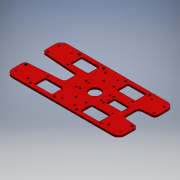
# Autodesk Inventor part: top_plate
Saved by Autodesk Inventor 2016 (Build 200138000, 138)
## iProperties
Created: 2015-12-08
Part Number: top_plate
Material: Generic
Document SubType Name: Modeling
Designer: lk8187
Density: 1 g/cm^3
Appearance: Smooth - Burnt Red
Author: lk8187
Autodesk Inventor part; units mm, degrees
ref_plane "YZ Plane" through (0, 0, 0) normal (1, 0, 0) x (0, 1, 0)
ref_plane "XZ Plane" through (0, 0, 0) normal (0, 1, 0) x (-1, 0, 0)
ref_plane "XY Plane" through (0, 0, 0) normal (0, 0, 1) x (1, 0, 0)
sketch "Sketch1" plane through (0, 0, 0) normal (0, 0, 1) x (1, 0, 0)
  line L0 (138.5, 75.5) -> (138.5, 61)
  arc A0 (136.5, 59) -> (138.5, 61) centre (136.5, 61) ccw
  line L1 (136.5, 59) -> (110, 59)
  arc A1 (108, 61) -> (110, 59) centre (110, 61) ccw
  line L2 (108, 61) -> (108, 75.5)
  arc A2 (110, 77.5) -> (108, 75.5) centre (110, 75.5) ccw
  line L3 (110, 77.5) -> (136.5, 77.5)
  arc A3 (138.5, 75.5) -> (136.5, 77.5) centre (136.5, 75.5) ccw
  line L4 (62, 75.5) -> (62, 61)
  arc A4 (60, 59) -> (62, 61) centre (60, 61) ccw
  line L5 (60, 59) -> (35, 59)
  arc A5 (33, 61) -> (35, 59) centre (35, 61) ccw
  line L6 (33, 61) -> (33, 75.5)
  arc A6 (35, 77.5) -> (33, 75.5) centre (35, 75.5) ccw
  line L7 (35, 77.5) -> (60, 77.5)
  arc A7 (62, 75.5) -> (60, 77.5) centre (60, 75.5) ccw
  line L8 (62, 17) -> (62, 2.5)
  arc A8 (60, 0.5) -> (62, 2.5) centre (60, 2.5) ccw
  line L9 (60, 0.5) -> (35, 0.5)
  arc A9 (33, 2.5) -> (35, 0.5) centre (35, 2.5) ccw
  line L10 (33, 2.5) -> (33, 17)
  arc A10 (35, 19) -> (33, 17) centre (35, 17) ccw
  line L11 (35, 19) -> (60, 19)
  arc A11 (62, 17) -> (60, 19) centre (60, 17) ccw
  line L12 (138.5, 17) -> (138.5, 2.5)
  arc A12 (136.5, 0.5) -> (138.5, 2.5) centre (136.5, 2.5) ccw
  line L13 (136.5, 0.5) -> (110, 0.5)
  arc A13 (108, 2.5) -> (110, 0.5) centre (110, 2.5) ccw
  line L14 (108, 2.5) -> (108, 17)
  arc A14 (110, 19) -> (108, 17) centre (110, 17) ccw
  line L15 (110, 19) -> (136.5, 19)
  arc A15 (138.5, 17) -> (136.5, 19) centre (136.5, 17) ccw
  arc A16 (176, 19.861) -> (171.3739, 24.847) centre (171, 19.861) ccw
  line L16 (171.3739, 24.847) -> (155.6261, 26.028)
  arc A17 (151, 31.014) -> (155.6261, 26.028) centre (156, 31.014) ccw
  line L17 (151, 31.014) -> (151, 46.986)
  arc A18 (155.6261, 51.972) -> (151, 46.986) centre (156, 46.986) ccw
  line L18 (155.6261, 51.972) -> (171.3739, 53.153)
  arc A19 (171.3739, 53.153) -> (176, 58.139) centre (171, 58.139) ccw
  line L19 (176, 58.139) -> (176, 73.5)
  arc A20 (176, 73.5) -> (166, 83.5) centre (166, 73.5) ccw
  line L20 (166, 83.5) -> (4, 83.5)
  arc A21 (4, 83.5) -> (-6, 73.5) centre (4, 73.5) ccw
  line L21 (-6, 73.5) -> (-6, 58.139)
  arc A22 (-6, 58.139) -> (-1.3739, 53.153) centre (-1, 58.139) ccw
  line L22 (-1.3739, 53.153) -> (49.3739, 49.347)
  arc A23 (54, 44.361) -> (49.3739, 49.347) centre (49, 44.361) ccw
  line L23 (54, 44.361) -> (54, 33.639)
  arc A24 (49.3739, 28.653) -> (54, 33.639) centre (49, 33.639) ccw
  line L24 (49.3739, 28.653) -> (-1.3739, 24.847)
  arc A25 (-1.3739, 24.847) -> (-6, 19.861) centre (-1, 19.861) ccw
  line L25 (-6, 19.861) -> (-6, 4.5)
  arc A26 (-6, 4.5) -> (4, -5.5) centre (4, 4.5) ccw
  line L26 (4, -5.5) -> (166, -5.5)
  arc A27 (166, -5.5) -> (176, 4.5) centre (166, 4.5) ccw
  line L27 (176, 4.5) -> (176, 19.861)
  line L28 (118.205, 45.5) -> (142.275, 45.5)
  line L29 (142.275, 45.5) -> (142.275, 32.5)
  line L30 (142.275, 32.5) -> (118.205, 32.5)
  line L31 (118.205, 32.5) -> (118.205, 45.5)
  circle A28 centre (150, 4) radius 1.5
  circle A29 centre (170, 74) radius 1.5
  circle A30 centre (75, 74) radius 1.5
  circle A31 centre (20, 74) radius 1.5
  circle A32 centre (0, 4) radius 1.5
  circle A33 centre (95, 4) radius 1.5
  circle A34 centre (0, 74) radius 1.5
  circle A35 centre (20, 4) radius 1.5
  circle A36 centre (75, 4) radius 1.5
  circle A37 centre (95, 74) radius 1.5
  circle A38 centre (150, 74) radius 1.5
  circle A39 centre (170, 4) radius 1.5
  circle A40 centre (93, 39) radius 9
  circle A41 centre (76, 32) radius 1.5
  circle A42 centre (76, 46) radius 1.5
  circle A43 centre (110, 32) radius 1.5
  circle A44 centre (110, 46) radius 1.5
  circle A45 centre (103, -0.5) radius 2
  circle A46 centre (67, 78.5) radius 2
  circle A47 centre (142, 78.5) radius 2
  circle A48 centre (67, -0.5) radius 2
  circle A49 centre (28, -0.5) radius 2
  circle A50 centre (142, -0.5) radius 2
  circle A51 centre (103, 78.5) radius 2
  circle A52 centre (28, 78.5) radius 2
  circle A53 centre (84.8683, 16.7261) radius 1.5
  circle A54 centre (115.2739, 30.8683) radius 1.5
  circle A55 centre (101.1317, 61.2739) radius 1.5
  circle A56 centre (70.7261, 47.1317) radius 1.5
  circle A57 centre (70.7261, 30.8683) radius 1.5
  circle A58 centre (84.8683, 61.2739) radius 1.5
  circle A59 centre (115.2739, 47.1317) radius 1.5
  circle A60 centre (101.1317, 16.7261) radius 1.5
  circle A61 centre (33, 55) radius 1.5
  circle A62 centre (138, 23) radius 1.5
  circle A63 centre (33, 23) radius 1.5
  circle A64 centre (138, 55) radius 1.5
  circle A65 centre (-1, 21) radius 2
  circle A66 centre (171, 57) radius 2
  circle A67 centre (171, 21) radius 2
  circle A68 centre (-1, 57) radius 2
  line L32 (93, 39) -> (118.205, 39) construction
  circle A69 centre (115.9525, 39) radius 1
  circle A70 centre (144.5275, 39) radius 1
  line L33 (144.5275, 39) -> (142.275, 39) construction
  line L34 (115.9525, 39) -> (118.205, 39) construction
  point P0 (0, 0)
  dimension "d2" = 4
  dimension "d3" = 8.578
  dimension "d4" = 25
  dimension "d5" = 6
  dimension "d6" = 6
  dimension "d7" = 6
  dimension "d8" = 6
  dimension "d9" = 24.07
  dimension "d10" = 13
  dimension "d11" = 2
  dimension "d12" = 33.725
  dimension "d13" = 28.575
  constraints: 71 centre point, 70 end point, 56 point on circle, 14 equal radius, 11 horizontal, 7 vertical, 4 tangent, 2 equal length, 2 midpoint, 145 other
  measures "d2" diameter of A52
  measures "d3" angle of L16 L18
  measures "d4" distance between parallel lines of L19 L17
  measures "d5" distance between parallel lines of L26 L9
  measures "d6" distance between parallel lines of L26 L13
  measures "d7" distance between parallel lines of L20 L3
  measures "d8" distance between parallel lines of L20 L7
  measures "d9" distance between parallel lines of L29 L31
  measures "d10" distance between parallel lines of L30 L28
  measures "d11" diameter of A69
  measures "d12" distance between parallel lines of L29 L19
  measures "d13" distance of L33.start L34.start
extrude "Extrusion1" add sketch "Sketch1" along normal blind 3
body "Solid1"
